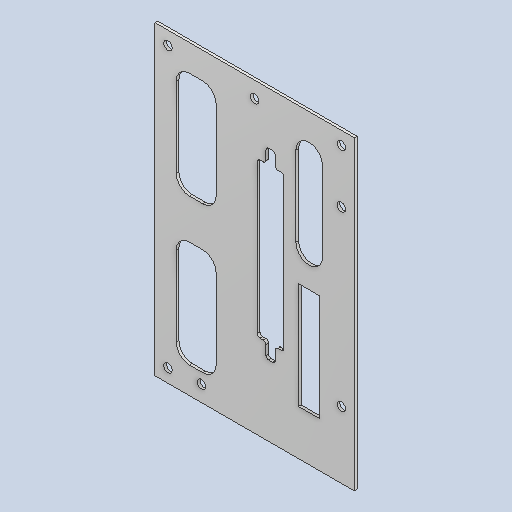
# Autodesk Inventor part: PCB_board_box_back
Saved by Autodesk Inventor 2023 (Build 270158000, 158)
## iProperties
Created: 2023-05-25
Part Number: PCB_board_box_back
Material: Aluminum
Document SubType Name: Sheet Metal
Designer: 310611102
Density: 2.7 g/cm^3
Sheet Metal Rule: 1mm
Appearance: Satin
Author: 310611102
Autodesk Inventor part; units mm, degrees
ref_plane "YZ Plane" through (0, 0, 0) normal (1, 0, 0) x (0, 1, 0)
ref_plane "XZ Plane" through (0, 0, 0) normal (0, 1, 0) x (-1, 0, 0)
ref_plane "XY Plane" through (0, 0, 0) normal (0, 0, 1) x (1, 0, 0)
sketch "Sketch1" plane through (0, 0, 0) normal (0, 0, 1) x (1, 0, 0)
  line L0 (-37.5, 57.5) -> (37.5, 57.5)
  line L1 (37.5, 57.5) -> (37.5, -57.5)
  line L2 (37.5, -57.5) -> (-37.5, -57.5)
  line L3 (-37.5, -57.5) -> (-37.5, 57.5)
  line L4 (-37.5, 57.5) -> (37.5, -57.5) construction
  line L5 (37.5, 57.5) -> (-37.5, -57.5) construction
  line L6 (11, 31.5) -> (11, -24.5)
  line L7 (1, -24.5) -> (1, 31.5)
  line L8 (1, 32.5) -> (11, -25.5) construction
  line L9 (11, 32.5) -> (1, -25.5) construction
  line L10 (5.25, 38) -> (6.75, 38)
  line L11 (7.75, 37) -> (7.75, 33.5)
  line L12 (4.25, 33.5) -> (4.25, 37)
  line L13 (4.25, 38) -> (7.75, 32.5) construction
  line L14 (7.75, 38) -> (4.25, 32.5) construction
  line L15 (5.25, -31) -> (6.75, -31)
  line L16 (7.75, -30) -> (7.75, -26.5)
  line L17 (4.25, -26.5) -> (4.25, -30)
  line L18 (4.25, -31) -> (7.75, -25.5) construction
  line L19 (7.75, -31) -> (4.25, -25.5) construction
  circle A0 centre (-32.6, 52.5) radius 1.6
  line L20 (0, 0) -> (0, 3.4669)
  line L21 (0, 0) -> (3.1568, 0)
  circle A1 centre (32.6, 52.5) radius 1.6
  circle A2 centre (-32.6, -52.5) radius 1.6
  circle A3 centre (-20, -51.5) radius 1.6
  circle A4 centre (32.6, -32.5) radius 1.6
  circle A5 centre (32.6, 32.5) radius 1.6
  circle A6 centre (0, 51.5) radius 1.6
  line L22 (16.5, -0.5) -> (24.5, -0.5)
  line L23 (24.5, -0.5) -> (24.5, -40.5)
  line L24 (24.5, -40.5) -> (16.5, -40.5)
  line L25 (16.5, -40.5) -> (16.5, -0.5)
  line L26 (16.5, -0.5) -> (24.5, -40.5) construction
  line L27 (24.5, -0.5) -> (16.5, -40.5) construction
  line L28 (-24.5, 47.5) -> (-19.5, 47.5)
  line L29 (-14.5, 42.5) -> (-14.5, 12.5)
  line L30 (-19.5, 7.5) -> (-24.5, 7.5)
  line L31 (-29.5, 12.5) -> (-29.5, 42.5)
  line L32 (-29.5, 47.5) -> (-14.5, 7.5) construction
  line L33 (-14.5, 47.5) -> (-29.5, 7.5) construction
  arc A7 (-24.5, 47.5) -> (-29.5, 42.5) centre (-24.5, 42.5) ccw
  arc A8 (-14.5, 42.5) -> (-19.5, 47.5) centre (-19.5, 42.5) ccw
  arc A9 (-19.5, 7.5) -> (-14.5, 12.5) centre (-19.5, 12.5) ccw
  arc A10 (-29.5, 12.5) -> (-24.5, 7.5) centre (-24.5, 12.5) ccw
  line L34 (-24.5, -47.5) -> (-19.5, -47.5)
  line L35 (-14.5, -42.5) -> (-14.5, -12.5)
  line L36 (-19.5, -7.5) -> (-24.5, -7.5)
  line L37 (-29.5, -12.5) -> (-29.5, -42.5)
  line L38 (-29.5, -47.5) -> (-14.5, -7.5) construction
  line L39 (-14.5, -47.5) -> (-29.5, -7.5) construction
  arc A11 (-29.5, -42.5) -> (-24.5, -47.5) centre (-24.5, -42.5) ccw
  arc A12 (-19.5, -47.5) -> (-14.5, -42.5) centre (-19.5, -42.5) ccw
  arc A13 (-14.5, -12.5) -> (-19.5, -7.5) centre (-19.5, -12.5) ccw
  arc A14 (-24.5, -7.5) -> (-29.5, -12.5) centre (-24.5, -12.5) ccw
  line L40 (20.5, 47.5) -> (20.5, 47.5)
  line L41 (25.5, 42.5) -> (25.5, 12.5)
  line L42 (20.5, 7.5) -> (20.5, 7.5)
  line L43 (15.5, 12.5) -> (15.5, 42.5)
  line L44 (15.5, 47.5) -> (25.5, 7.5) construction
  line L45 (25.5, 47.5) -> (15.5, 7.5) construction
  arc A15 (20.5, 47.5) -> (15.5, 42.5) centre (20.5, 42.5) ccw
  arc A16 (25.5, 42.5) -> (20.5, 47.5) centre (20.5, 42.5) ccw
  arc A17 (20.5, 7.5) -> (25.5, 12.5) centre (20.5, 12.5) ccw
  arc A18 (15.5, 12.5) -> (20.5, 7.5) centre (20.5, 12.5) ccw
  arc A19 (5.25, 38) -> (4.25, 37) centre (5.25, 37) ccw
  arc A20 (7.75, 37) -> (6.75, 38) centre (6.75, 37) ccw
  arc A21 (4.25, -30) -> (5.25, -31) centre (5.25, -30) ccw
  arc A22 (6.75, -31) -> (7.75, -30) centre (6.75, -30) ccw
  line L46 (10, -25.5) -> (8.75, -25.5)
  line L47 (3.25, -25.5) -> (2, -25.5)
  line L48 (2, 32.5) -> (3.25, 32.5)
  line L49 (8.75, 32.5) -> (10, 32.5)
  arc A23 (2, 32.5) -> (1, 31.5) centre (2, 31.5) ccw
  arc A24 (3.25, 32.5) -> (4.25, 33.5) centre (3.25, 33.5) ccw
  arc A25 (7.75, 33.5) -> (8.75, 32.5) centre (8.75, 33.5) ccw
  arc A26 (11, 31.5) -> (10, 32.5) centre (10, 31.5) ccw
  arc A27 (10, -25.5) -> (11, -24.5) centre (10, -24.5) ccw
  arc A28 (8.75, -25.5) -> (7.75, -26.5) centre (8.75, -26.5) ccw
  arc A29 (4.25, -26.5) -> (3.25, -25.5) centre (3.25, -26.5) ccw
  arc A30 (1, -24.5) -> (2, -25.5) centre (2, -24.5) ccw
  point P0 (6, 3.5)
  point P1 (6, 35.25)
  point P2 (6, -28.25)
  point P3 (20.5, -20.5)
  point P4 (-22, 27.5)
  point P5 (-22, -27.5)
  point P6 (20.5, 27.5)
  point P7 (0, -57.5)
  point P8 (0, 57.5)
  dimension "d0" = 75
  dimension "d1" = 115
  dimension "d2" = 3.5
  dimension "d3" = 5.5
  dimension "d4" = 10
  dimension "d5" = 58
  dimension "d6" = 26.5
  dimension "d9" = 3.2
  dimension "d10" = 5
  dimension "d11" = 4.9
  dimension "d14" = 3.2
  dimension "d15" = 6
  dimension "d16" = 3.2
  dimension "d18" = 4.9
  dimension "d19" = 25
  dimension "d20" = 8
  dimension "d21" = 40
  dimension "d23" = 13
  dimension "d24" = 17
  dimension "d25" = 15
  dimension "d26" = 40
  dimension "d27" = 5
  dimension "d28" = 10
  dimension "d29" = 8
  dimension "d30" = 40
  dimension "d31" = 10
  dimension "d32" = 12
  dimension "d33" = 10
  dimension "d34" = 5
  dimension "d36" = 20
  dimension "d37" = 6
  dimension "d38" = 0
  dimension "d39" = 3.2
  dimension "d40" = 1
  dimension "d41" = 25
  dimension "d42" = 1
  measures "d0" distance of L0.start L0.end
  measures "d1" distance of L0.end L1.end
  measures "d2" distance of L13.start L14.start
  measures "d3" distance of L14.start L13.end
  measures "d4" distance of L8.start L9.start
  measures "d5" distance of L9.end L8.start
  measures "d6" distance between parallel lines of L1 L6
  measures "d9" diameter of A0
  measures "d10" distance from line of L0 A0.centre
  measures "d11" distance from line of A0.centre L3
  measures "d14" diameter of A3
  measures "d15" distance from line of L2 A3.centre
  measures "d16" diameter of A4
  measures "d18" distance from line of L1 A4.centre
  measures "d19" distance from line of L2 A4.centre
  measures "d20" distance of L22.start L22.end
  measures "d21" distance of L22.end L23.end
  measures "d23" distance between parallel lines of L1 L23
  measures "d24" distance between parallel lines of L2 L24
  measures "d25" distance of L32.start L33.start
  measures "d26" distance of L33.end L32.start
  measures "d27" radius of A7
  measures "d28" distance between parallel lines of L0 L28
  measures "d29" distance between parallel lines of L3 L31
  measures "d30" distance between parallel lines of L42 L40
  measures "d31" distance of L44.end L45.end
  measures "d32" distance between parallel lines of L1 L41
  measures "d33" distance between parallel lines of L0 L40
  measures "d34" radius of A15
  measures "d36" horizontal distance of point (0, -57.5) A3.centre
  measures "d37" distance from line of L0 A6.centre
  measures "d38" horizontal distance of point (0, 57.5) A6.centre
  measures "d39" diameter of A6
  measures "d40" radius of A19
  measures "d41" distance between parallel lines of L0 L48
  measures "d42" radius of A23
extrude "Plate1" add sketch "Sketch1" along normal blind 1
equation "\"d8\" = 厚度"
equation "\"折彎半徑\" = 厚度"
equation "\"折彎離隙寬度\" = 厚度"
equation "\"折彎離隙深度\" = 0.5 * 厚度"
equation "\"轉角離隙大小\" = 4 * 厚度"
equation "\"最小剩餘\" = 2 * 厚度"
equation "\"轉移半徑\" = 折彎半徑"
equation "\"Jacobi半徑大小\" = 折彎半徑"
equation "\"間隙大小\" = 厚度"
equation "\"厚度\" = 1"
body "Solid1"
